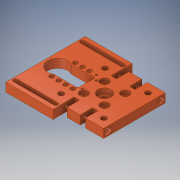
# Autodesk Inventor part: КВ33.044.901 - Щека каретки Z
Saved by Autodesk Inventor 2019 (Build 230136000, 136)
## iProperties
Created: 2019-08-08
Part Number: КВ33.044.901 - Щека каретки Z
Material: Пластик АБС
Document SubType Name: Modeling
Designer: user
Density: 1.06 g/cm^3
Appearance: Гладкий — светло-оранжевый
Author: user
Autodesk Inventor part; units mm, degrees
ref_plane "YZ Plane" through (0, 0, 0) normal (1, 0, 0) x (0, 1, 0)
ref_plane "XZ Plane" through (0, 0, 0) normal (0, 1, 0) x (-1, 0, 0)
ref_plane "XY Plane" through (0, 0, 0) normal (0, 0, 1) x (1, 0, 0)
sketch "Эскиз4" plane through (0, 0, 0) normal (0, 1, 0) x (-1, 0, 0)
  circle A0 centre (-24.3, 25) radius 3
  circle A1 centre (24.3, 25) radius 3
  circle A2 centre (24.3, -25) radius 3
  circle A3 centre (-24.3, -25) radius 3
  line L0 (13.5, -21) -> (13.5, -35)
  line L1 (13.5, -35) -> (34, -35)
  line L2 (34, -35) -> (34, 35)
  line L3 (34, 35) -> (13.5, 35)
  line L4 (13.5, 35) -> (13.5, 21)
  line L5 (13.5, 21) -> (7.5, 21)
  line L6 (7.5, 21) -> (7.5, 35)
  line L7 (7.5, 35) -> (-7.5, 35)
  line L8 (-7.5, 35) -> (-7.5, 21)
  line L9 (-7.5, 21) -> (-13.5, 21)
  line L10 (-13.5, 21) -> (-13.5, 35)
  line L11 (-13.5, 35) -> (-34, 35)
  line L12 (-34, 35) -> (-34, -35)
  line L13 (-34, -35) -> (-13.5, -35)
  line L14 (-13.5, -35) -> (-13.5, -21)
  line L15 (-13.5, -21) -> (-7.5, -21)
  line L16 (-7.5, -21) -> (-7.5, -35)
  line L17 (-7.5, -35) -> (7.5, -35)
  line L18 (7.5, -35) -> (7.5, -21)
  line L19 (7.5, -21) -> (13.5, -21)
  circle A4 centre (0, 0) radius 7.5
  circle A5 centre (-11.75, 11.7501) radius 4.65
  circle A6 centre (-11.7501, -11.75) radius 4.65
  line L20 (26, 12) -> (16.3934, 12)
  line L21 (26, -12) -> (26, 12)
  line L22 (16.3933, -12) -> (26, -12)
  arc A7 (16, -9.8634) -> (16.3933, -12) centre (11.75, -11.7501) ccw
  line L23 (16, -9.8634) -> (16, 9.8629)
  arc A8 (16.3934, 12) -> (16, 9.8629) centre (11.7501, 11.75) ccw
  circle A9 centre (-11.75, 11.7501) radius 2.6
  circle A10 centre (-11.7501, -11.75) radius 2.6
  circle A11 centre (11.75, -11.7501) radius 2.6
  circle A12 centre (11.7501, 11.75) radius 2.6
  circle A13 centre (0, 0) radius 4.1
  circle A14 centre (11.7501, 11.75) radius 4.65
  circle A15 centre (11.75, -11.7501) radius 4.65
  constraints: 48 end point, 14 centre point, 4 point on circle, 2 coincident, 6 other
extrude "Выдавливание3" add sketch "Эскиз4" along normal blind 10 contours L19 L18 L17 L16 L15 L14 L13 L12 L11 L10 L9 L8 L7 L6 L5 L4 L3 L2 L1 L0 | A4 | A5 | A6 | L21 L22 A15 L23 A14 L20 | A14 A8 | A7 A15
sketch "Эскиз5" plane through (0, 10, 0) normal (0, 1, 0) x (1, 0, 0)
  circle A0 centre (-24.3, 25) radius 3
  circle A1 centre (24.3, 25) radius 3
  circle A2 centre (24.3, -25) radius 3
  circle A3 centre (-24.3, -25) radius 3
  line L0 (13.5, -21) -> (13.5, -35)
  line L1 (13.5, -35) -> (34, -35)
  line L2 (34, -35) -> (34, 35)
  line L3 (34, 35) -> (13.5, 35)
  line L4 (13.5, 35) -> (13.5, 21)
  line L5 (13.5, 21) -> (7.5, 21)
  line L6 (7.5, 21) -> (7.5, 35)
  line L7 (7.5, 35) -> (-7.5, 35)
  line L8 (-7.5, 35) -> (-7.5, 21)
  line L9 (-7.5, 21) -> (-13.5, 21)
  line L10 (-13.5, 21) -> (-13.5, 35)
  line L11 (-13.5, 35) -> (-34, 35)
  line L12 (-34, 35) -> (-34, -35)
  line L13 (-34, -35) -> (-13.5, -35)
  line L14 (-13.5, -35) -> (-13.5, -21)
  line L15 (-13.5, -21) -> (-7.5, -21)
  line L16 (-7.5, -21) -> (-7.5, -35)
  line L17 (-7.5, -35) -> (7.5, -35)
  line L18 (7.5, -35) -> (7.5, -21)
  line L19 (7.5, -21) -> (13.5, -21)
  circle A4 centre (0, 0) radius 7.5
  circle A5 centre (-11.75, 11.7501) radius 4.65
  circle A6 centre (-11.7501, -11.75) radius 4.65
  line L20 (26, 12) -> (16.3934, 12)
  line L21 (26, -12) -> (26, 12)
  line L22 (16.3933, -12) -> (26, -12)
  arc A7 (16, -9.8634) -> (16.3933, -12) centre (11.75, -11.7501) ccw
  line L23 (16, -9.8634) -> (16, 9.8629)
  arc A8 (16.3934, 12) -> (16, 9.8629) centre (11.7501, 11.75) ccw
  circle A9 centre (-11.75, 11.7501) radius 2.6
  circle A10 centre (-11.7501, -11.75) radius 2.6
  circle A11 centre (11.75, -11.7501) radius 2.6
  circle A12 centre (11.7501, 11.75) radius 2.6
  circle A13 centre (0, 0) radius 4.1
  circle A14 centre (11.75, -11.7501) radius 2.6 projected
  circle A15 centre (11.75, -11.7501) radius 4.65
  circle A16 centre (11.7501, 11.75) radius 4.65
  constraints: 48 end point, 16 centre point, 4 point on circle, 2 coincident, 2 concentric
extrude "Выдавливание4" cut sketch "Эскиз5" against normal blind 4 contours A5 | A6 | A16 A8 | A7 A15
sketch "Эскиз6" plane through (0, 10, 0) normal (0, 1, 0) x (1, 0, 0)
  circle A0 centre (-24.3, 25) radius 3
  circle A1 centre (24.3, 25) radius 3
  circle A2 centre (24.3, -25) radius 3
  circle A3 centre (-24.3, -25) radius 3
  line L0 (13.5, -21) -> (13.5, -35)
  line L1 (13.5, -35) -> (34, -35)
  line L2 (34, -35) -> (34, 35)
  line L3 (34, 35) -> (13.5, 35)
  line L4 (13.5, 35) -> (13.5, 21)
  line L5 (13.5, 21) -> (7.5, 21)
  line L6 (7.5, 21) -> (7.5, 35)
  line L7 (7.5, 35) -> (-7.5, 35)
  line L8 (-7.5, 35) -> (-7.5, 21)
  line L9 (-7.5, 21) -> (-13.5, 21)
  line L10 (-13.5, 21) -> (-13.5, 35)
  line L11 (-13.5, 35) -> (-34, 35)
  line L12 (-34, 35) -> (-34, -35)
  line L13 (-34, -35) -> (-13.5, -35)
  line L14 (-13.5, -35) -> (-13.5, -21)
  line L15 (-13.5, -21) -> (-7.5, -21)
  line L16 (-7.5, -21) -> (-7.5, -35)
  line L17 (-7.5, -35) -> (7.5, -35)
  line L18 (7.5, -35) -> (7.5, -21)
  line L19 (7.5, -21) -> (13.5, -21)
  circle A4 centre (0, 0) radius 7.5
  circle A5 centre (-11.75, 11.7501) radius 4.65
  circle A6 centre (-11.7501, -11.75) radius 4.65
  line L20 (26, 12) -> (16.3934, 12)
  line L21 (26, -12) -> (26, 12)
  line L22 (16.3933, -12) -> (26, -12)
  arc A7 (16, -9.8634) -> (16.3933, -12) centre (11.75, -11.7501) ccw
  line L23 (16, -9.8634) -> (16, 9.8629)
  arc A8 (16.3934, 12) -> (16, 9.8629) centre (11.7501, 11.75) ccw
  circle A9 centre (-11.75, 11.7501) radius 2.6
  circle A10 centre (-11.7501, -11.75) radius 2.6
  circle A11 centre (11.75, -11.7501) radius 2.6
  circle A12 centre (11.7501, 11.75) radius 2.6
  circle A13 centre (0, 0) radius 4.1
  constraints: 48 end point, 14 centre point, 4 point on circle
extrude "Выдавливание5" cut sketch "Эскиз6" against normal blind 6 contours A4
sketch "Эскиз7" plane through (34, 0, 35) normal (1, 0, 0) x (0, 0, -1)
  circle A0 centre (5, 5) radius 2
  circle A1 centre (5, 5) radius 4
  circle A2 centre (65, 5) radius 4
  circle A3 centre (5, 5) radius 4
  line L0 (0, 0) -> (70, 0)
  line L1 (70, 0) -> (70, 10)
  line L2 (0, 10) -> (70, 10)
  line L3 (0, 0) -> (0, 10)
  circle A4 centre (65, 5) radius 2
  circle A5 centre (65, 5) radius 4
  point P0 (35, 0)
  point P1 (35, 0)
  constraints: 8 end point, 6 centre point
extrude "Выдавливание6" cut sketch "Эскиз7" against normal blind 269 contours A0 | A4
sketch "Эскиз8" plane through (34, 0, 35) normal (1, 0, 0) x (0, 0, -1)
  circle A0 centre (5, 5) radius 2
  circle A1 centre (5, 5) radius 4
  circle A2 centre (65, 5) radius 4
  circle A3 centre (5, 5) radius 4
  line L0 (0, 0) -> (70, 0)
  line L1 (70, 0) -> (70, 10)
  line L2 (0, 10) -> (70, 10)
  line L3 (0, 0) -> (0, 10)
  circle A4 centre (65, 5) radius 2
  circle A5 centre (65, 5) radius 4
  point P0 (35, 0)
  point P1 (35, 0)
  constraints: 8 end point, 6 centre point
extrude "Выдавливание7" cut sketch "Эскиз8" against normal blind 15 contours A1 | A2
sketch "Эскиз9" plane through (-34, 0, -35) normal (-1, 0, 0) x (0, 0, 1)
  circle A0 centre (5, 5) radius 2
  circle A1 centre (5, 5) radius 4
  circle A2 centre (65, 5) radius 4
  circle A3 centre (5, 5) radius 4
  line L0 (0, 0) -> (70, 0)
  line L1 (70, 0) -> (70, 10)
  line L2 (0, 10) -> (70, 10)
  line L3 (0, 0) -> (0, 10)
  circle A4 centre (65, 5) radius 2
  circle A5 centre (65, 5) radius 4
  point P0 (35, 0)
  point P1 (35, 0)
  constraints: 8 end point, 6 centre point
extrude "Выдавливание8" cut sketch "Эскиз9" against normal blind 15 contours A1 | A2
sketch "Эскиз17" plane through (-34, 0, -35) normal (-1, 0, 0) x (0, 0, 1)
  line L0 (14, 10) -> (0, 10) projected
  line L1 (70, 0) -> (56, 0) projected
  line L2 (0, 10) -> (70, 10)
  line L3 (70, 10) -> (70, 0)
  line L4 (70, 0) -> (0, 0)
  line L5 (0, 0) -> (0, 10)
  point P0 (35, 0)
  constraints: 8 end point, 2 parallel, 1 horizontal, 1 perpendicular
extrude "Выдавливание14" add sketch "Эскиз17" along normal blind 33
sketch "Эскиз18" plane through (0, 0, 0) normal (0, -1, 0) x (1, 0, 0)
  line L0 (-35.2, -12.6) -> (-35.2, -14.9)
  line L1 (-35.2, -12.6) -> (-33.8, -12.6)
  line L2 (-33.8, -14.9) -> (-33.8, -12.6)
  line L3 (-27.2, -14.9) -> (-33.8, -14.9)
  line L4 (-27.2, -12.6) -> (-27.2, -14.9)
  circle A0 centre (-53, 0) radius 9.15
  circle A1 centre (-53, 0) radius 1.5
  circle A2 centre (-17, 8) radius 1.3
  circle A3 centre (-30.5, 13.5) radius 1.3
  circle A4 centre (-22.5, 13.5) radius 1.3
  circle A5 centre (-38.5, 13.5) radius 1.3
  circle A6 centre (-46.5, 13.5) radius 1.3
  circle A7 centre (-17, -8) radius 1.3
  circle A8 centre (-30.5, -13.5) radius 1.3
  circle A9 centre (-22.5, -13.5) radius 1.3
  circle A10 centre (-38.5, -13.5) radius 1.3
  circle A11 centre (-46.5, -13.5) radius 1.3
  line L5 (-64.0198, -0.1) -> (-63.4796, -0.1)
  line L6 (-64.0198, -7) -> (-64.0198, -0.1)
  arc A12 (-64.0198, -7) -> (-63.9686, -7.75) centre (-58.5, -7) ccw
  line L7 (-61.5, -7.75) -> (-63.9686, -7.75)
  arc A13 (-59.75, -9.5) -> (-61.5, -7.75) centre (-61.5, -9.5) ccw
  line L8 (-59.75, -10) -> (-59.75, -9.5)
  line L9 (-22.1937, -10) -> (-59.75, -10)
  arc A14 (-22.1937, -10) -> (-21.5055, -9.6078) centre (-22.1937, -9.2) ccw
  arc A15 (-21.5055, -9.6078) -> (-20.8922, -8.9945) centre (-20, -10.5) ccw
  arc A16 (-20.8922, -8.9945) -> (-20.5, -8.3063) centre (-21.3, -8.3063) ccw
  line L10 (-20.5, 8.3063) -> (-20.5, -8.3063)
  arc A17 (-20.5, 8.3063) -> (-20.8922, 8.9945) centre (-21.3, 8.3063) ccw
  arc A18 (-21.5055, 9.6078) -> (-20.8922, 8.9945) centre (-20, 10.5) ccw
  arc A19 (-20.8922, 8.9945) -> (-21.5055, 9.6078) centre (-20, 10.5) ccw
  line L11 (-59.75, -11.3229) -> (-59.75, -10)
  arc A20 (-59.75, -11.3229) -> (-58.5, -11.5) centre (-58.4989, -6.9922) ccw
  line L12 (-58.5, -11.5) -> (-51, -11.5)
  line L13 (-51, -12.6) -> (-51, -11.5)
  line L14 (-49.8, -12.6) -> (-51, -12.6)
  line L15 (-49.8, -14.9) -> (-49.8, -12.6)
  line L16 (-43.2, -14.9) -> (-49.8, -14.9)
  line L17 (-43.2, -12.6) -> (-43.2, -14.9)
  line L18 (-41.8, -12.6) -> (-43.2, -12.6)
  line L19 (-41.8, -14.9) -> (-41.8, -12.6)
  line L20 (-35.2, -14.9) -> (-41.8, -14.9)
  line L21 (-35.2, -12.6) -> (-35.2, -14.9)
  line L22 (-33.8, -12.6) -> (-35.2, -12.6)
  line L23 (-33.8, -14.9) -> (-33.8, -12.6)
  line L24 (-27.2, -14.9) -> (-33.8, -14.9)
  line L25 (-27.2, -12.6) -> (-27.2, -14.9)
  line L26 (-25.8, -12.6) -> (-27.2, -12.6)
  line L27 (-25.8, -14.9) -> (-25.8, -12.6)
  line L28 (-19.2, -14.9) -> (-25.8, -14.9)
  line L29 (-19.2, -12.6) -> (-19.2, -14.9)
  line L30 (-17.9802, -12.6) -> (-19.2, -12.6)
  arc A21 (-17.9802, -12.6) -> (-17.9, -12.5198) centre (-19, -11.5) ccw
  line L31 (-17.9, -11.3) -> (-17.9, -12.5198)
  line L32 (-15.6, -11.3) -> (-17.9, -11.3)
  line L33 (-15.6, -4.7) -> (-15.6, -11.3)
  line L34 (-17.9, -4.7) -> (-15.6, -4.7)
  line L35 (-17.9, 4.7) -> (-17.9, -4.7)
  line L36 (-15.6, 4.7) -> (-17.9, 4.7)
  line L37 (-15.6, 11.3) -> (-15.6, 4.7)
  line L38 (-17.9, 11.3) -> (-15.6, 11.3)
  line L39 (-17.9, 12.5198) -> (-17.9, 11.3)
  arc A22 (-17.9, 12.5198) -> (-17.9802, 12.6) centre (-19, 11.5) ccw
  line L40 (-19.2, 12.6) -> (-17.9802, 12.6)
  line L41 (-19.2, 14.9) -> (-19.2, 12.6)
  line L42 (-25.8, 14.9) -> (-19.2, 14.9)
  line L43 (-25.8, 12.6) -> (-25.8, 14.9)
  line L44 (-27.2, 12.6) -> (-25.8, 12.6)
  line L45 (-27.2, 14.9) -> (-27.2, 12.6)
  line L46 (-33.8, 14.9) -> (-27.2, 14.9)
  line L47 (-33.8, 12.6) -> (-33.8, 14.9)
  line L48 (-35.2, 12.6) -> (-33.8, 12.6)
  line L49 (-35.2, 14.9) -> (-35.2, 12.6)
  line L50 (-41.8, 14.9) -> (-35.2, 14.9)
  line L51 (-41.8, 12.6) -> (-41.8, 14.9)
  line L52 (-43.2, 12.6) -> (-41.8, 12.6)
  line L53 (-43.2, 14.9) -> (-43.2, 12.6)
  line L54 (-49.8, 14.9) -> (-43.2, 14.9)
  line L55 (-49.8, 12.6) -> (-49.8, 14.9)
  line L56 (-51, 12.6) -> (-49.8, 12.6)
  line L57 (-51, 11.5) -> (-51, 12.6)
  line L58 (-58.5, 11.5) -> (-51, 11.5)
  arc A23 (-58.5, 11.5) -> (-59.75, 11.3229) centre (-58.4989, 6.9922) ccw
  line L59 (-59.75, 10) -> (-59.75, 11.3229)
  line L60 (-59.75, 9.5) -> (-59.75, 10)
  arc A24 (-61.5, 7.75) -> (-59.75, 9.5) centre (-61.5, 9.5) ccw
  line L61 (-63.9686, 7.75) -> (-61.5, 7.75)
  arc A25 (-63.9686, 7.75) -> (-64.0198, 7) centre (-58.5, 7) ccw
  line L62 (-64.0198, 0.1) -> (-64.0198, 7)
  line L63 (-63.4796, 0.1) -> (-64.0198, 0.1)
  arc A26 (-20.8922, -8.9945) -> (-21.5055, -9.6078) centre (-20, -10.5) ccw
  arc A27 (-21.5055, 9.6078) -> (-22.1937, 10) centre (-22.1937, 9.2) ccw
  line L64 (-59.75, 10) -> (-22.1937, 10)
  line L65 (0, 0) -> (-34, 0)
  line L66 (-34, 0) -> (-53, 0)
  line L67 (-53, -9.15) -> (-53, -10)
  line L68 (-53, 10) -> (-53, 9.15)
  dimension "d62" = 34
  dimension "d63" = 19
  constraints: 138 end point, 34 point on circle, 28 centre point, 4 point on line, 2 horizontal, 1 perpendicular
  measures "d62" distance of L65.start L65.end
  measures "d63" distance of L65.end L66.end
extrude "Выдавливание15" cut sketch "Эскиз18" against normal blind 23 contours L67 A0 L66 L65 L10 A16 A26 A14 L9 | A0 | L68 L64 A27 A18 A17 L10 L65 L66 A0 | A1 | A2 | A3 | A4 | A5 | A6 | A7 | A8 | A9 | A10 | A11
sketch "Эскиз19" plane through (0, 0, 0) normal (0, -1, 0) x (1, 0, 0)
  arc A0 (-53, 9.15) -> (-53, -9.15) centre (-53, 0) ccw projected
  circle A1 centre (-53, 0) radius 11.5
  point P0 (0, 0)
  dimension "d66" = 23
  constraints: 1 centre point, 1 coincident
  measures "d66" diameter of A1
extrude "Выдавливание16" cut sketch "Эскиз19" against normal blind 23
sketch "Эскиз20" plane through (0, 10, 0) normal (0, 1, 0) x (1, 0, 0)
  circle A0 centre (-22.5, -13.5) radius 1.3 projected
  circle A1 centre (-22.5, -13.5) radius 2.5
  circle A2 centre (-30.5, -13.5) radius 1.3 projected
  circle A3 centre (-30.5, -13.5) radius 2.5
  circle A4 centre (-38.5, -13.5) radius 1.3 projected
  circle A5 centre (-38.5, -13.5) radius 2.5
  circle A6 centre (-46.5, -13.5) radius 1.3 projected
  circle A7 centre (-46.5, -13.5) radius 2.5
  circle A8 centre (-46.5, 13.5) radius 1.3 projected
  circle A9 centre (-46.5, 13.5) radius 2.5
  circle A10 centre (-38.5, 13.5) radius 1.3 projected
  circle A11 centre (-38.5, 13.5) radius 2.5
  circle A12 centre (-30.5, 13.5) radius 1.3 projected
  circle A13 centre (-30.5, 13.5) radius 2.5
  circle A14 centre (-22.5, 13.5) radius 1.3 projected
  circle A15 centre (-22.5, 13.5) radius 2.5
  point P0 (0, 0)
  dimension "d69" = 5
  dimension "d70" = 5
  dimension "d71" = 5
  dimension "d72" = 5
  dimension "d73" = 5
  dimension "d74" = 5
  dimension "d75" = 5
  dimension "d76" = 5
  constraints: 8 centre point, 8 coincident
  measures "d69" diameter of A1
  measures "d70" diameter of A3
  measures "d71" diameter of A5
  measures "d72" diameter of A7
  measures "d73" diameter of A9
  measures "d74" diameter of A11
  measures "d75" diameter of A13
  measures "d76" diameter of A15
extrude "Выдавливание17" cut sketch "Эскиз20" against normal blind 2 contours A0 | A1 | A2 | A3 | A4 | A5 | A6 | A7 | A8 | A9 | A10 | A11 | A12 | A13 | A14
move faces "Перенос3" translate (0, 0, -10) faces at (-49.1667, 6.6667, -35)
move faces "Перенос4" translate (0, 0, 10) faces at (-31.3333, 6.6667, 35)
sketch "Эскиз21" plane through (0, 10, 0) normal (0, 1, 0) x (1, 0, 0)
  line L0 (-13.5, -45) -> (-67, -45) projected
  line L1 (-40.25, -45) -> (-40.25, -38)
  line L2 (-13.5, 45) -> (-67, 45) projected
  line L3 (-40.25, 45) -> (-40.25, 38)
  line L4 (-17.1684, -38) -> (-63.3316, -38) construction
  line L5 (-17.1684, -35.75) -> (-63.3316, -35.75)
  line L6 (-63.3316, -40.25) -> (-17.1684, -40.25)
  arc A0 (-17.1684, -40.25) -> (-17.1684, -35.75) centre (-17.1684, -38) ccw
  arc A1 (-63.3316, -35.75) -> (-63.3316, -40.25) centre (-63.3316, -38) ccw
  line L7 (-17.1684, 38) -> (-63.3316, 38) construction
  line L8 (-17.1684, 40.25) -> (-63.3316, 40.25)
  line L9 (-63.3316, 35.75) -> (-17.1684, 35.75)
  arc A2 (-17.1684, 35.75) -> (-17.1684, 40.25) centre (-17.1684, 38) ccw
  arc A3 (-63.3316, 40.25) -> (-63.3316, 35.75) centre (-63.3316, 38) ccw
  point P0 (0, 0)
  dimension "d85" = 7
  dimension "d86" = 7
  dimension "d87" = 90
  dimension "d88" = 4.5
  dimension "d89" = 4.5
  constraints: 20 end point, 8 point on circle, 8 tangent, 4 centre point, 4 midpoint, 2 horizontal, 2 parallel, 1 vertical
  measures "d85" distance of L1.start L1.end
  measures "d86" distance of L3.start L3.end
  measures "d87" angle of L2 L3
  measures "d88" diameter of A1
  measures "d89" diameter of A3
extrude "Выдавливание18" cut sketch "Эскиз21" against normal blind 15.5
